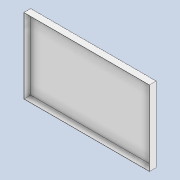
# Autodesk Inventor part: Tapa_superior_derecha
Saved by Autodesk Inventor 2021 (Build 250183000, 183)
## iProperties
Created: 2021-04-15
Part Number: Tapa_superior_derecha
Material: Genérico
Document SubType Name: Modeling
Designer: Admin
Density: 1 g/cm^3
Appearance: Blanco
Author: Admin
Autodesk Inventor part; units mm, degrees
ref_plane "YZ Plane" through (0, 0, 0) normal (1, 0, 0) x (0, 1, 0)
ref_plane "XZ Plane" through (0, 0, 0) normal (0, 1, 0) x (-1, 0, 0)
ref_plane "XY Plane" through (0, 0, 0) normal (0, 0, 1) x (1, 0, 0)
sketch "Boceto1" plane through (0, 0, 0) normal (0, 0, 1) x (1, 0, 0)
  line L0 (0, 0) -> (385, 0)
  line L1 (385, 0) -> (385, 230)
  line L2 (385, 230) -> (0, 230)
  line L3 (0, 230) -> (0, 0)
  dimension "d0" = 385
  dimension "d1" = 230
  constraints: 8 end point, 2 parallel, 1 horizontal, 1 perpendicular
  measures "d0" distance of L2.end L1.end
  measures "d1" distance of L1.end L0.end
extrude "Extrusión1" add sketch "Boceto1" along normal blind 0.76
sketch "Boceto2" plane through (0, 0, 0.76) normal (0, 0, 1) x (1, 0, 0)
  line L0 (385, 230) -> (0, 230) projected
  line L1 (0, 0) -> (0.76, 0)
  line L2 (0.76, 0.76) -> (0.76, 229.24)
  line L3 (0.76, 230) -> (0, 230)
  line L4 (0, 230) -> (0, 0)
  line L5 (0, 230) -> (0, 0) projected
  line L6 (385, 0) -> (385, 230) projected
  line L7 (0, 0) -> (385, 0)
  line L8 (385, 0) -> (385, 0.76)
  line L9 (384.24, 0.76) -> (0.76, 0.76)
  line L10 (0, 0.76) -> (0, 0)
  line L11 (0, 0) -> (385, 0) projected
  line L12 (385, 0) -> (384.24, 0)
  line L13 (384.24, 0.76) -> (384.24, 229.24)
  line L14 (384.24, 230) -> (385, 230)
  line L15 (385, 230) -> (385, 0)
  line L16 (385, 230) -> (0, 230)
  line L17 (0, 230) -> (0, 229.24)
  line L18 (0.76, 229.24) -> (384.24, 229.24)
  line L19 (385, 229.24) -> (385, 230)
  dimension "d4" = 0.76
  dimension "d5" = 0.76
  dimension "d6" = 0.76
  dimension "d7" = 0.76
  constraints: 32 end point, 8 parallel, 4 horizontal, 4 perpendicular, 4 point on line
  measures "d4" distance of L3.end L3.start
  measures "d5" distance of L8.end L7.end
  measures "d6" distance of L14.start L14.end
  measures "d7" distance of L17.end L16.end
extrude "Extrusión2" add sketch "Boceto2" along normal blind 20
